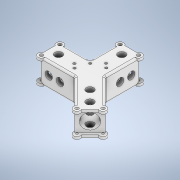
# Autodesk Inventor part: BracketV3
Saved by Autodesk Inventor 2022 (Build 260153000, 153)
## iProperties
Created: 2022-02-09
Part Number: BracketV3
Material: Generic
Document SubType Name: Modeling
Designer: ultra
Density: 1 g/cm^3
Appearance: Smooth - White
Author: ultra
Autodesk Inventor part; units mm, degrees
ref_plane "YZ Plane" through (0, 0, 0) normal (1, 0, 0) x (0, 1, 0)
ref_plane "XZ Plane" through (0, 0, 0) normal (0, 1, 0) x (-1, 0, 0)
ref_plane "XY Plane" through (0, 0, 0) normal (0, 0, 1) x (1, 0, 0)
sketch "Sketch1" plane through (0, 0, 0) normal (1, 0, 0) x (0, 1, 0)
  line L0 (0, 0) -> (41.5544, 0)
  line L1 (41.5544, 0) -> (41.5544, 37.0078)
  line L2 (41.5544, 37.0078) -> (0, 37.0078)
  line L3 (0, 37.0078) -> (0, 0)
  circle A0 centre (20.7772, 18.5039) radius 12.8778
  dimension "d0" = 41.5544
  dimension "d1" = 37.0078
  dimension "d2" = 25.7556
  constraints: 8 end point, 2 parallel, 1 centre point, 1 horizontal, 1 perpendicular
  measures "d0" distance of L2.end L1.end
  measures "d1" distance of L1.end L0.end
  measures "d2" diameter of A0
extrude "Extrusion1" add sketch "Sketch1" along normal blind 50.8
sketch "Sketch2" plane through (0, 0, 0) normal (0, 0, -1) x (-1, 0, 0)
  line L0 (-50.8, 0) -> (-50.8, 41.5544) projected
  line L1 (-50.8, 41.5544) -> (-87.8078, 41.5544)
  line L2 (-87.8078, 41.5544) -> (-87.8078, 0)
  line L3 (-87.8078, 0) -> (-50.8, 0)
  line L4 (-50.8, 0) -> (-50.8, 41.5544)
  circle A0 centre (-69.3039, 20.7772) radius 12.8778
  dimension "d5" = 37.0078
  dimension "d6" = 25.7556
  constraints: 8 end point, 2 parallel, 1 centre point, 1 horizontal, 1 perpendicular
  measures "d5" distance of L3.end L2.end
  measures "d6" diameter of A0
extrude "Extrusion2" add sketch "Sketch2" against normal up to surface (37.0078 mm away) contours L3 L2 L1 L0 | A0
sketch "Sketch3" plane through (0, 0, 0) normal (0, 0, -1) x (-1, 0, 0)
  line L0 (0, 41.5544) -> (-87.8078, 41.5544) projected
  line L1 (-87.8078, 41.5544) -> (-87.8078, 0) projected
  line L2 (0, 0) -> (-87.8078, 0) projected
  line L3 (0, 0) -> (-87.8078, 0) projected
  line L4 (-87.8078, 41.5544) -> (-50.8, 41.5544)
  line L5 (-50.8, 41.5544) -> (-50.8, 0)
  line L6 (-50.8, 0) -> (-87.8078, 0)
  line L7 (-87.8078, 0) -> (-87.8078, 41.5544)
  circle A0 centre (-69.3039, 20.7772) radius 12.8778
  point P0 (-50.8, 0)
  dimension "d9" = 37.0078
  dimension "d10" = 25.7556
  constraints: 8 end point, 2 parallel, 1 centre point, 1 horizontal, 1 perpendicular, 1 point on line
  measures "d9" distance of L5.end L6.end
  measures "d10" diameter of A0
extrude "Extrusion3" add sketch "Sketch3" along normal blind 50.8
sketch "Sketch4" plane through (0, 41.5544, 37.0078) normal (0, 1, 0) x (1, 0, 0)
  line L0 (0, 0) -> (87.8078, 0) projected
  line L1 (87.8078, 87.8078) -> (87.8078, 0) projected
  line L2 (50.8, 37.0078) -> (50.8, 87.8078) projected
  line L3 (87.8078, 0) -> (87.8078, 87.8078) projected
  line L4 (50.8, 37.0078) -> (87.8078, 0)
  line L5 (87.8078, 0) -> (123.1594, -36.4815)
  line L6 (87.8078, 0) -> (100.892, 13.0842)
  line L7 (0, 0) -> (87.8078, 0) projected
  line L8 (87.8078, 0) -> (74.7236, -13.0842)
  line L9 (100.892, 13.0842) -> (87.8078, 26.1685)
  line L10 (74.7236, -13.0842) -> (61.6393, 0)
  line L11 (100.892, 13.0842) -> (136.8086, -22.8323)
  line L12 (136.8086, -22.8323) -> (123.1594, -36.4815)
  line L13 (123.1594, -36.4815) -> (110.6401, -49.0008)
  line L14 (123.1594, -36.4815) -> (140.8643, -36.4815) construction
  line L15 (110.6401, -49.0008) -> (74.7236, -13.0842)
  dimension "d13" = 50.8
  dimension "d14" = 18.5039
  dimension "d15" = 18.5039
  dimension "d16" = 135
  constraints: 22 end point, 4 point on line, 3 perpendicular, 1 equal length, 1 horizontal
  measures "d13" distance of L0.end L5.end
  measures "d14" distance of L0.end L6.end
  measures "d15" distance of L0.end L8.end
  measures "d16" angle of L13 L14
extrude "Extrusion4" add sketch "Sketch4" against normal up to surface (41.5544 mm away)
sketch "Sketch5" plane through (136.8086, 0, 59.8401) normal (0.7071068, 0, 0.7071068) x (0.7071068, 0, -0.7071068)
  line L0 (-18.5039, 41.5544) -> (-18.5039, 0) projected
  circle A0 centre (-18.5039, 20.7772) radius 12.8778
  point P0 (-54.4249, 0)
  dimension "d19" = 25.7556
  constraints: 1 centre point, 1 midpoint
  measures "d19" diameter of A0
extrude "Extrusion5" cut sketch "Sketch5" against normal blind 76.2
sketch "Sketch6" plane through (0, 41.5544, 37.0078) normal (0, 1, 0) x (1, 0, 0)
  line L0 (0, 37.0078) -> (0, 0) projected
  line L1 (0, 0) -> (61.6393, 0) projected
  line L2 (61.6393, 0) -> (110.6401, -49.0008) projected
  line L3 (110.6401, -49.0008) -> (136.8086, -22.8323) projected
  line L4 (136.8086, -22.8323) -> (87.8078, 26.1685) projected
  line L5 (87.8078, 87.8078) -> (87.8078, 26.1685) projected
  line L6 (50.8, 87.8078) -> (87.8078, 87.8078) projected
  line L7 (50.8, 37.0078) -> (50.8, 87.8078) projected
  line L8 (0, 37.0078) -> (50.8, 37.0078) projected
  line L9 (0, 18.5039) -> (69.3039, 18.5039)
  line L10 (69.3039, 18.5039) -> (69.3039, 87.8078)
  line L11 (56.4261, 87.8078) -> (82.1817, 87.8078) projected
  line L12 (69.3039, 18.5039) -> (123.7244, -35.9166)
  circle A0 centre (2.4892, 2.879) radius 1.778
  circle A1 centre (2.4892, 34.1288) radius 1.778
  circle A2 centre (84.9288, 85.3186) radius 1.778
  circle A3 centre (53.679, 85.3186) radius 1.778
  circle A4 centre (110.9158, -45.2049) radius 1.778
  circle A5 centre (133.0127, -23.108) radius 1.778
  dimension "d22" = 3.556
  dimension "d23" = 3.556
  dimension "d24" = 2.4892
  dimension "d25" = 2.4892
  dimension "d26" = 2.879
  dimension "d27" = 2.879
  dimension "d28" = 3.556
  dimension "d29" = 3.556
  dimension "d30" = 2.4892
  dimension "d31" = 2.4892
  dimension "d32" = 2.879
  dimension "d33" = 2.879
  dimension "d34" = 3.556
  dimension "d35" = 3.556
  dimension "d36" = 2.4892
  dimension "d37" = 2.4892
  dimension "d38" = 2.879
  dimension "d39" = 2.879
  constraints: 6 centre point, 6 end point, 3 midpoint, 1 perpendicular
  measures "d22" diameter of A0
  measures "d23" diameter of A1
  measures "d24" distance from line of L0 A0.centre
  measures "d25" distance from line of L0 A1.centre
  measures "d26" distance from line of L1 A0.centre
  measures "d27" distance from line of L8 A1.centre
  measures "d28" diameter of A2
  measures "d29" diameter of A3
  measures "d30" vertical distance of L11.start A3.centre
  measures "d31" distance from line of L6 A2.centre
  measures "d32" distance from line of L5 A2.centre
  measures "d33" distance from line of L7 A3.centre
  measures "d34" diameter of A4
  measures "d35" diameter of A5
  measures "d36" distance from line of L3 A4.centre
  measures "d37" distance from line of L3 A5.centre
  measures "d38" distance from line of L4 A5.centre
  measures "d39" distance from line of L2 A4.centre
extrude "Extrusion6" cut sketch "Sketch6" against normal blind 50.8 contours A0 | A1 | A2 | A3 | A4 | A5
sketch "Sketch7" plane through (0, 41.5544, 37.0078) normal (0, 1, 0) x (1, 0, 0)
  circle A0 centre (2.4892, 2.879) radius 1.778 projected
  circle A1 centre (110.9158, -45.2049) radius 1.778 projected
  circle A2 centre (53.679, 85.3186) radius 1.778 projected
  circle A3 centre (2.4892, 34.1288) radius 1.778 projected
  circle A4 centre (84.9288, 85.3186) radius 1.778 projected
  line L0 (0, 37.0078) -> (0, 0) projected
  line L1 (0, 0) -> (61.6393, 0) projected
  line L2 (61.6393, 0) -> (110.6401, -49.0008) projected
  line L3 (110.6401, -49.0008) -> (136.8086, -22.8323) projected
  line L4 (136.8086, -22.8323) -> (87.8078, 26.1685) projected
  line L5 (87.8078, 87.8078) -> (87.8078, 26.1685) projected
  line L6 (50.8, 87.8078) -> (87.8078, 87.8078) projected
  line L7 (50.8, 37.0078) -> (50.8, 87.8078) projected
  line L8 (0, 37.0078) -> (50.8, 37.0078) projected
  circle A5 centre (133.0127, -23.108) radius 1.778 projected
  circle A6 centre (133.0127, -23.108) radius 6
  circle A7 centre (110.9158, -45.2049) radius 6
  circle A8 centre (2.4892, 2.879) radius 6
  circle A9 centre (2.4892, 34.1288) radius 6
  circle A10 centre (53.679, 85.3186) radius 6
  circle A11 centre (84.9288, 85.3186) radius 6
  point P0 (0, 8.3383)
  point P1 (7.7534, 0)
  point P2 (7.7534, 37.0078)
  point P3 (0, 28.6695)
  point P4 (59.1383, 87.8078)
  point P5 (50.8, 80.0544)
  point P6 (79.4695, 87.8078)
  point P7 (87.8078, 80.0544)
  point P8 (130.9126, -28.7284)
  point P9 (131.3262, -17.3499)
  point P10 (105.1577, -43.5184)
  point P11 (116.5362, -43.1048)
  dimension "d42" = 12
  dimension "d43" = 12
  dimension "d44" = 12
  dimension "d45" = 12
  dimension "d46" = 12
  dimension "d47" = 12
  constraints: 6 centre point, 6 coincident
  measures "d42" diameter of A6
  measures "d43" diameter of A7
  measures "d44" diameter of A8
  measures "d45" diameter of A9
  measures "d46" diameter of A10
  measures "d47" diameter of A11
extrude "Extrusion7" add sketch "Sketch7" against normal blind 4.7752 contours L0 A9 L8 | L0 L1 A8 | A10 L6 L7 | L2 L3 A7 | A11 L5 L6 | L3 L4 A6 picked at (-0.4033, 31.694) picked at (-0.4033, 5.3138) picked at (56.1138, 88.2111) picked at (106.9061, -45.8277) picked at (82.5067, 88.2271) picked at (133.3453, -26.876)
sketch "Sketch8" plane through (0, 0, 0) normal (0, -1, 0) x (1, 0, 0)
  circle A0 centre (2.4892, 34.1288) radius 1.778 projected
  circle A1 centre (53.679, -48.3108) radius 1.778 projected
  circle A2 centre (2.4892, 2.879) radius 1.778 projected
  circle A3 centre (84.9288, -48.3108) radius 1.778 projected
  line L0 (0, 37.0078) -> (0, 0) projected
  line L1 (0, 0) -> (50.8, 0) projected
  line L2 (50.8, 0) -> (50.8, -50.8) projected
  line L3 (87.8078, -50.8) -> (50.8, -50.8) projected
  line L4 (87.8078, 10.8393) -> (87.8078, -50.8) projected
  line L5 (136.8086, 59.8401) -> (87.8078, 10.8393) projected
  line L6 (110.6401, 86.0086) -> (136.8086, 59.8401) projected
  line L7 (61.6393, 37.0078) -> (110.6401, 86.0086) projected
  line L8 (0, 37.0078) -> (61.6393, 37.0078) projected
  circle A4 centre (110.9158, 82.2127) radius 1.778 projected
  circle A5 centre (110.9158, 82.2127) radius 6
  circle A6 centre (133.0127, 60.1158) radius 1.778 projected
  circle A7 centre (133.0127, 60.1158) radius 6
  circle A8 centre (84.9288, -48.3108) radius 6
  circle A9 centre (53.679, -48.3108) radius 6
  circle A10 centre (2.4892, 2.879) radius 6
  circle A11 centre (2.4892, 34.1288) radius 6
  point P0 (0, 8.3383)
  point P1 (7.7534, 0)
  point P2 (7.7534, 37.0078)
  point P3 (0, 28.6695)
  point P4 (116.5362, 80.1126)
  point P5 (105.1577, 80.5262)
  point P6 (131.3262, 54.3577)
  point P7 (130.9126, 65.7362)
  point P8 (87.8078, -43.0466)
  point P9 (79.4695, -50.8)
  point P10 (50.8, -43.0466)
  point P11 (59.1383, -50.8)
  dimension "d50" = 12
  constraints: 6 centre point, 6 coincident
  measures "d50" diameter of A5
extrude "Extrusion8" add sketch "Sketch8" against normal blind 4.7752 contours L0 A11 L8 | L0 L1 A10 | A5 L6 L7 | L2 L3 A9 | A7 L5 L6 | L3 L4 A8 picked at (-0.4033, 31.694) picked at (-0.4033, 5.3138) picked at (106.9061, 82.8355) picked at (56.1138, -51.2033) picked at (133.3453, 63.8838) picked at (82.5067, -51.2193)
sketch "Sketch9" plane through (0, 41.5544, 28.6695) normal (0, 1, 0) x (1, 0, 0)
  circle A0 centre (2.4892, -5.4593) radius 1.778 projected
  circle A1 centre (110.9158, -53.5432) radius 1.778 projected
  circle A2 centre (53.679, 76.9803) radius 1.778 projected
  circle A3 centre (2.4892, 25.7905) radius 1.778 projected
  circle A4 centre (133.0127, -31.4463) radius 1.778 projected
  circle A5 centre (84.9288, 76.9803) radius 1.778 projected
  arc A6 (0, 0) -> (7.7534, -8.3383) centre (2.4892, -5.4593) ccw projected
  arc A7 (105.1577, -51.8567) -> (116.5362, -51.443) centre (110.9158, -53.5432) ccw projected
  arc A8 (87.8078, 71.7161) -> (79.4695, 79.4695) centre (84.9288, 76.9803) ccw projected
  arc A9 (7.7534, 28.6695) -> (0, 20.3312) centre (2.4892, 25.7905) ccw projected
  circle A10 centre (110.9158, -53.5432) radius 2.95
  circle A11 centre (133.0127, -31.4463) radius 1.778 projected
  circle A12 centre (133.0127, -31.4463) radius 2.95
  circle A13 centre (84.9288, 76.9803) radius 2.95
  circle A14 centre (53.679, 76.9803) radius 1.778 projected
  circle A15 centre (53.679, 76.9803) radius 2.95
  circle A16 centre (2.4892, 25.7905) radius 2.95
  circle A17 centre (2.4892, -5.4593) radius 2.95
  point P0 (0, 28.6695)
  dimension "d53" = 5.9
  dimension "d54" = 5.9
  dimension "d55" = 5.9
  dimension "d56" = 5.9
  dimension "d57" = 5.9
  dimension "d58" = 5.9
  constraints: 6 centre point, 6 coincident
  measures "d53" diameter of A10
  measures "d54" diameter of A12
  measures "d55" diameter of A13
  measures "d56" diameter of A15
  measures "d57" diameter of A16
  measures "d58" diameter of A17
sketch "Sketch10" plane through (0, 0, -50.8) normal (0, 0, -1) x (-1, 0, 0)
  line L0 (-59.1383, 4.7752) -> (-50.8, 4.7752) projected
  line L1 (-50.8, 4.7752) -> (-50.8, 36.7792) projected
  line L2 (-50.8, 36.7792) -> (-59.1383, 36.7792) projected
  line L3 (-79.4695, 36.7792) -> (-87.8078, 36.7792) projected
  line L4 (-87.8078, 36.7792) -> (-87.8078, 4.7752) projected
  line L5 (-87.8078, 4.7752) -> (-79.4695, 4.7752) projected
  circle A0 centre (-69.3039, 20.7772) radius 12.8778 projected
  line L6 (-87.8078, 4.7752) -> (-50.8, 4.7752)
  line L7 (-50.8, 4.7752) -> (-50.8, 36.7792)
  line L8 (-50.8, 36.7792) -> (-87.8078, 36.7792)
  line L9 (-87.8078, 36.7792) -> (-87.8078, 4.7752)
  line L10 (-87.8078, 4.7752) -> (-50.8, 36.7792) construction
  line L11 (-50.8, 4.7752) -> (-87.8078, 36.7792) construction
  point P0 (0, 0)
  constraints: 12 end point, 2 midpoint, 2 parallel, 1 horizontal, 1 perpendicular
extrude "Extrusion9" cut sketch "Sketch10" against normal blind 5.0038
sketch "Sketch11" plane through (0, 0, 0) normal (-1, 0, 0) x (0, 0, 1)
  line L0 (28.6695, 4.7752) -> (37.0078, 4.7752) projected
  line L1 (37.0078, 36.7792) -> (37.0078, 4.7752) projected
  line L2 (37.0078, 36.7792) -> (28.6695, 36.7792) projected
  line L3 (8.3383, 36.7792) -> (0, 36.7792) projected
  line L4 (0, 4.7752) -> (0, 36.7792) projected
  line L5 (0, 4.7752) -> (8.3383, 4.7752) projected
  circle A0 centre (18.5039, 20.7772) radius 12.8778 projected
  line L6 (0, 4.7752) -> (37.0078, 4.7752)
  line L7 (37.0078, 4.7752) -> (37.0078, 36.7792)
  line L8 (37.0078, 36.7792) -> (0, 36.7792)
  line L9 (0, 36.7792) -> (0, 4.7752)
  line L10 (0, 4.7752) -> (37.0078, 36.7792) construction
  line L11 (37.0078, 4.7752) -> (0, 36.7792) construction
  point P0 (0, 0)
  constraints: 12 end point, 2 midpoint, 2 parallel, 1 horizontal, 1 perpendicular
extrude "Extrusion10" cut sketch "Sketch11" against normal blind 5.0038
sketch "Sketch12" plane through (130.9126, 36.7792, 65.7362) normal (0.7071068, 0, 0.7071068) x (0.7071068, 0, -0.7071068)
  line L0 (0, -32.004) -> (8.3383, -32.004) projected
  line L1 (8.3383, 0) -> (8.3383, -32.004) projected
  line L2 (8.3383, 0) -> (0, 0) projected
  line L3 (-20.3312, 0) -> (-28.6695, 0) projected
  line L4 (-28.6695, 0) -> (-28.6695, -32.004) projected
  line L5 (-28.6695, -32.004) -> (-20.3312, -32.004) projected
  circle A0 centre (-10.1656, -16.002) radius 12.8778 projected
  line L6 (-28.6695, -32.004) -> (8.3383, -32.004)
  line L7 (8.3383, -32.004) -> (8.3383, 0)
  line L8 (8.3383, 0) -> (-28.6695, 0)
  line L9 (-28.6695, 0) -> (-28.6695, -32.004)
  line L10 (-28.6695, -32.004) -> (8.3383, 0) construction
  line L11 (8.3383, -32.004) -> (-28.6695, 0) construction
  point P0 (-46.0866, -36.7792)
  point P1 (-20.3312, 0)
  point P2 (-20.3312, -32.004)
  constraints: 12 end point, 2 midpoint, 2 parallel, 1 horizontal, 1 perpendicular
extrude "Extrusion11" cut sketch "Sketch12" against normal blind 5.0038
extrude "Extrusion12" cut sketch "Sketch9" against normal blind 5.08
fillet "Fillet1" radius 3.175 15 edges at (50.8, 20.7772, 0) (29.2767, 41.5544, 0) (50.8, 41.5544, -21.5233) (50.8, 0, -21.5233) (29.2767, 0, 0) (34.6963, 41.5544, 37.0078) (83.3985, 41.5544, 58.767) (83.3985, 0, 58.767) (109.567, 41.5544, 32.5985) (109.567, 0, 32.5985) (87.8078, 41.5544, -16.1037) (87.8078, 0, -16.1037) (34.6963, 0, 37.0078) (61.6393, 20.7772, 37.0078) (87.8078, 20.7772, 10.8393)
sketch "Sketch15" plane through (0, 0, 8.3383) normal (0, -1, 0) x (1, 0, 0)
  line L0 (0, 0) -> (0, 20.3312) projected
  line L1 (116.755, -37.314) -> (68.3935, 11.0475)
  line L2 (68.3935, 11.0475) -> (118.0223, 60.6763)
  line L3 (68.3935, 11.0475) -> (18.7646, 60.6763) construction
  line L4 (73.5122, 12.7537) -> (70.0997, 16.1662)
  line L5 (70.0997, 16.1662) -> (63.2747, 9.3412)
  line L6 (63.2747, 9.3412) -> (66.6872, 5.9287)
  line L7 (66.6872, 5.9287) -> (73.5122, 12.7537)
  line L8 (73.5122, 12.7537) -> (63.2747, 9.3412) construction
  line L9 (70.0997, 16.1662) -> (66.6872, 5.9287) construction
  line L10 (78.0024, 12.7537) -> (70.0997, 20.6564)
  line L11 (70.0997, 20.6564) -> (58.7846, 9.3412)
  line L12 (58.7846, 9.3412) -> (66.6872, 1.4386)
  line L13 (66.6872, 1.4386) -> (78.0024, 12.7537)
  line L14 (78.0024, 12.7537) -> (58.7846, 9.3412) construction
  line L15 (70.0997, 20.6564) -> (66.6872, 1.4386) construction
  point P0 (0, -8.3383)
  dimension "d104" = 90
  dimension "d105" = 4.826
  dimension "d106" = 9.652
  dimension "d107" = 11.176
  dimension "d108" = 16.002
  constraints: 30 end point, 4 midpoint, 4 parallel, 3 perpendicular
  measures "d104" angle of L2 L3
  measures "d105" distance of L6.end L5.end
  measures "d106" distance of L5.end L4.end
  measures "d107" distance of L12.end L11.end
  measures "d108" distance of L11.end L10.end
extrude "Extrusion14" add sketch "Sketch15" along normal blind 12.7 contours L13 L12 L11 L10 L2 L4 L5 L6 L7 L1 | L1 L7 L4 L2 L10 L13
sketch "Sketch16" plane through (58.7846, 0, 17.6795) normal (-0.7071068, 0, 0.7071068) x (0.7071068, 0, 0.7071068)
  line L0 (0, 0) -> (0, -12.7) projected
  line L1 (16.002, -12.7) -> (0, -12.7) projected
  circle A0 centre (8.001, -7.112) radius 3.175
  point P0 (-54.0683, 0)
  dimension "d111" = 6.35
  dimension "d112" = 8.001
  dimension "d113" = 5.588
  constraints: 1 centre point
  measures "d111" diameter of A0
  measures "d112" distance from line of L0 A0.centre
  measures "d113" distance from line of A0.centre L1
extrude "Extrusion15" cut sketch "Sketch16" against normal blind 279.4
sketch "Sketch18" plane through (0, 41.5544, 28.6695) normal (0, 1, 0) x (1, 0, 0)
  circle A0 centre (76.2759, 30.7551) radius 2.159
  circle A1 centre (69.4016, 37.3483) radius 2.159
  circle A2 centre (55.9312, 23.8779) radius 2.159
  circle A3 centre (42.7448, 10.1294) radius 2.159
  circle A4 centre (49.6191, 3.5362) radius 2.159
  point P0 (0, 28.6695)
  dimension "d149" = 4.318
  dimension "d150" = 4.318
  dimension "d151" = 4.318
  dimension "d152" = 4.318
  dimension "d153" = 4.318
  constraints: 5 centre point
  measures "d149" diameter of A0
  measures "d150" diameter of A1
  measures "d151" diameter of A2
  measures "d152" diameter of A3
  measures "d153" diameter of A4
fillet "Fillet2" radius 6.35 4 edges at (62.7359, 0, 13.7282) (72.3448, 0, 15.4345) (74.051, 0, 25.0433) (64.4422, 0, 23.3371)
fillet "Fillet3" radius 3.175 8 edges at (66.6872, -1.8599, 7.1467) (66.6872, -9.525, 9.7769) (80.6326, -1.8599, 21.092) (78.0024, -9.525, 21.092) (70.0997, -1.8599, 31.6249) (70.0997, -9.525, 28.9947) (56.1544, -1.8599, 17.6795) (58.7846, -9.525, 17.6795)
sketch "Sketch20" plane through (0, 36.7792, 37.0078) normal (0, -1, 0) x (1, 0, 0)
  arc A0 (5.0038, -1.3365) -> (5.0038, -4.4215) centre (2.4892, -2.879) ccw projected
  line L0 (5.0038, -1.3365) -> (5.0038, 0) projected
  line L1 (7.7534, 0) -> (5.0038, 0) projected
  arc A1 (7.7534, 0) -> (0, -8.3383) centre (2.4892, -2.879) ccw projected
  line L2 (0, -28.6695) -> (0, -8.3383) projected
  arc A2 (0, -28.6695) -> (7.7534, -37.0078) centre (2.4892, -34.1288) ccw projected
  line L3 (5.0038, -37.0078) -> (7.7534, -37.0078) projected
  line L4 (5.0038, -37.0078) -> (5.0038, -35.6713) projected
  arc A3 (5.0038, -32.5863) -> (5.0038, -35.6713) centre (2.4892, -34.1288) ccw projected
  line L5 (5.0038, -32.5863) -> (5.0038, -4.4215) projected
  point P0 (0, -37.0078)
extrude "Extrusion19" cut sketch "Sketch20" against normal blind 0.381
sketch "Sketch21" plane through (0, 4.7752, 0) normal (0, 1, 0) x (1, 0, 0)
  circle A0 centre (2.4892, -34.1288) radius 1.5875 projected
  circle A1 centre (2.4892, -2.879) radius 1.5875 projected
  line L0 (7.7534, 0) -> (5.0038, 0) projected
  arc A2 (7.7534, 0) -> (0, -8.3383) centre (2.4892, -2.879) ccw projected
  line L1 (0, -28.6695) -> (0, -8.3383) projected
  arc A3 (0, -28.6695) -> (7.7534, -37.0078) centre (2.4892, -34.1288) ccw projected
  line L2 (5.0038, -37.0078) -> (7.7534, -37.0078) projected
  line L3 (5.0038, -37.0078) -> (5.0038, 0) projected
  point P0 (0, 0)
extrude "Extrusion20" cut sketch "Sketch21" against normal blind 0.381
sketch "Sketch22" plane through (0, 4.7752, 0) normal (0, 1, 0) x (1, 0, 0)
  circle A0 centre (53.679, 48.3108) radius 1.5875 projected
  circle A1 centre (84.9288, 48.3108) radius 1.5875 projected
  line L0 (87.8078, 43.0466) -> (87.8078, 45.7962) projected
  arc A2 (87.8078, 43.0466) -> (79.4695, 50.8) centre (84.9288, 48.3108) ccw projected
  line L1 (59.1383, 50.8) -> (79.4695, 50.8) projected
  arc A3 (59.1383, 50.8) -> (50.8, 43.0466) centre (53.679, 48.3108) ccw projected
  line L2 (50.8, 45.7962) -> (50.8, 43.0466) projected
  line L3 (50.8, 45.7962) -> (87.8078, 45.7962) projected
  point P0 (0, 0)
extrude "Extrusion21" cut sketch "Sketch22" against normal blind 0.381
sketch "Sketch23" plane through (0, 4.7752, 0) normal (0, 1, 0) x (1, 0, 0)
  circle A0 centre (110.9158, -82.2127) radius 1.5875 projected
  circle A1 centre (133.0127, -60.1158) radius 1.5875 projected
  line L0 (105.1577, -80.5262) -> (107.1019, -82.4704) projected
  arc A2 (105.1577, -80.5262) -> (116.5362, -80.1126) centre (110.9158, -82.2127) ccw projected
  line L1 (130.9126, -65.7362) -> (116.5362, -80.1126) projected
  arc A3 (130.9126, -65.7362) -> (131.3262, -54.3577) centre (133.0127, -60.1158) ccw projected
  line L2 (133.2704, -56.3019) -> (131.3262, -54.3577) projected
  line L3 (133.2704, -56.3019) -> (107.1019, -82.4704) projected
  point P0 (0, 0)
extrude "Extrusion22" cut sketch "Sketch23" against normal blind 0.381
sketch "Sketch24" plane through (0, 36.7792, 37.0078) normal (0, -1, 0) x (1, 0, 0)
  arc A0 (52.1365, -82.804) -> (55.2215, -82.804) centre (53.679, -85.3186) ccw projected
  line L0 (52.1365, -82.804) -> (50.8, -82.804) projected
  line L1 (50.8, -80.0544) -> (50.8, -82.804) projected
  arc A1 (50.8, -80.0544) -> (59.1383, -87.8078) centre (53.679, -85.3186) ccw projected
  line L2 (79.4695, -87.8078) -> (59.1383, -87.8078) projected
  arc A2 (79.4695, -87.8078) -> (87.8078, -80.0544) centre (84.9288, -85.3186) ccw projected
  line L3 (87.8078, -82.804) -> (87.8078, -80.0544) projected
  line L4 (87.8078, -82.804) -> (86.4713, -82.804) projected
  arc A3 (83.3863, -82.804) -> (86.4713, -82.804) centre (84.9288, -85.3186) ccw projected
  line L5 (83.3863, -82.804) -> (55.2215, -82.804) projected
  point P0 (0, -37.0078)
extrude "Extrusion23" cut sketch "Sketch24" against normal blind 0.381
sketch "Sketch25" plane through (0, 36.7792, 37.0078) normal (0, -1, 0) x (1, 0, 0)
  arc A0 (110.2284, 42.3361) -> (108.047, 44.5175) centre (110.9158, 45.2049) ccw projected
  line L0 (110.2284, 42.3361) -> (130.1439, 22.4206) projected
  arc A1 (132.3253, 20.2392) -> (130.1439, 22.4206) centre (133.0127, 23.108) ccw projected
  line L1 (132.3253, 20.2392) -> (133.2704, 19.2941) projected
  line L2 (131.3262, 17.3499) -> (133.2704, 19.2941) projected
  arc A2 (131.3262, 17.3499) -> (130.9126, 28.7284) centre (133.0127, 23.108) ccw projected
  line L3 (116.5362, 43.1048) -> (130.9126, 28.7284) projected
  arc A3 (116.5362, 43.1048) -> (105.1577, 43.5184) centre (110.9158, 45.2049) ccw projected
  line L4 (107.1019, 45.4626) -> (105.1577, 43.5184) projected
  line L5 (107.1019, 45.4626) -> (108.047, 44.5175) projected
  point P0 (0, -37.0078)
extrude "Extrusion24" cut sketch "Sketch25" against normal blind 0.381
extrude "Extrusion25" cut sketch "Sketch18" against normal blind 9.525
sketch "Sketch27" plane through (62.5693, 3.175, 37.9377) normal (-0.7071068, 0, 0.7071068) x (0.7071068, 0, 0.7071068)
  line L0 (62.9787, 1.2192) -> (62.9787, 33.9852) projected
  line L1 (0, 0) -> (0, 35.2044) projected
  line L2 (62.9787, 33.9852) -> (62.9787, 1.2192) projected
  line L3 (62.9787, 17.6022) -> (0, 17.6022)
  circle A0 centre (50.2787, 17.6022) radius 6.35
  circle A1 centre (24.8787, 17.6022) radius 6.35
  point P0 (-71.0692, -3.175)
  dimension "d162" = 12.7
  dimension "d163" = 12.7
  dimension "d166" = 25.4
  constraints: 2 centre point, 2 end point, 2 midpoint, 1 horizontal, 1 point on line, 2 other
  measures "d162" diameter of A0
  measures "d163" distance from line of L0 A0.centre
  measures "d166" distance of A0.centre A1.centre
extrude "Extrusion27" cut sketch "Sketch27" against normal blind 76.2
sketch "Sketch28" plane through (7.7534, 3.175, 37.0078) normal (0, 0, 1) x (1, 0, 0)
  line L0 (52.5708, 35.2044) -> (52.5708, 0) projected
  line L1 (-2.7496, 33.9852) -> (-2.7496, 1.2192) projected
  line L2 (-2.7496, 30.48) -> (-2.7496, 4.7244) projected
  line L3 (-2.7496, 17.6022) -> (52.9835, 17.6022)
  ellipse E0 centre (62.0895, 17.6022) end of major axis (62.0895, 4.7244) minor radius 9.106 projected
  circle A0 centre (9.9504, 17.6022) radius 6.35
  circle A1 centre (29.0004, 17.6022) radius 6.35
  point P0 (-7.7534, -3.175)
  dimension "d173" = 12.7
  dimension "d174" = 12.7
  dimension "d177" = 19.05
  constraints: 2 centre point, 2 end point, 1 horizontal, 1 horizontal alignment, 1 midpoint, 1 perpendicular, 1 point on line, 3 other
  measures "d173" diameter of A0
  measures "d174" distance from line of L1 A0.centre
  measures "d177" distance of A0.centre A1.centre
extrude "Extrusion28" cut sketch "Sketch28" against normal blind 76.2 contours A0 L3 | L3 A0 | A1 L3 | L3 A1
sketch "Sketch29" plane through (50.8, 3.175, -3.175) normal (-1, 0, 0) x (0, 0, 1)
  line L0 (0, 0) -> (-39.8716, 0) projected
  line L1 (-42.6212, 33.9852) -> (-42.6212, 1.2192) projected
  circle A0 centre (-29.9212, 17.6022) radius 6.35
  circle A1 centre (-10.8712, 17.6022) radius 6.35
  point P0 (3.175, -3.175)
  dimension "d184" = 12.7
  dimension "d185" = 12.7
  dimension "d188" = 19.05
  constraints: 2 centre point, 1 horizontal, 2 other
  measures "d184" diameter of A0
  measures "d185" distance from line of L1 A0.centre
  measures "d188" distance of A0.centre A1.centre
extrude "Extrusion29" cut sketch "Sketch29" against normal blind 76.2
sketch "Sketch31" plane through (0, 41.5544, 28.6695) normal (0, 1, 0) x (1, 0, 0)
  line L0 (53.975, 31.8445) -> (53.975, 70.9876) projected
  arc A0 (47.625, 25.4945) -> (53.975, 31.8445) centre (47.625, 31.8445) ccw projected
  line L1 (0, 20.3312) -> (0, 0) projected
  line L2 (116.5362, -51.443) -> (130.9126, -37.0667) projected
  line L3 (123.7244, -44.2549) -> (52.1151, 27.3544)
  line L4 (79.4695, 79.4695) -> (59.1383, 79.4695) projected
  line L5 (69.3039, 79.4695) -> (69.3039, 10.1656)
  line L6 (69.3039, 10.1656) -> (0, 10.1656)
  line L7 (69.3039, 79.4695) -> (69.3039, 66.7695)
  line L8 (69.3039, 66.7695) -> (76.9747, 66.7695)
  line L9 (69.3039, 66.7695) -> (61.6331, 66.7695)
  circle A1 centre (76.9747, 66.7695) radius 2.54
  circle A2 centre (61.6331, 66.7695) radius 2.54
  circle A3 centre (61.6331, 47.7195) radius 2.54
  circle A4 centre (76.9747, 47.7195) radius 2.54
  line L10 (123.7244, -44.2549) -> (114.7441, -35.2746)
  line L11 (114.7441, -35.2746) -> (120.1682, -29.8505)
  line L12 (120.1682, -29.8505) -> (114.7441, -35.2746)
  line L13 (114.7441, -35.2746) -> (109.3201, -40.6987)
  line L14 (0, 10.1656) -> (12.7, 10.1656)
  line L15 (12.7, 10.1656) -> (12.7, 2.4948)
  line L16 (12.7, 2.4948) -> (12.7, 10.1656)
  line L17 (12.7, 10.1656) -> (12.7, 17.8364)
  circle A5 centre (12.7, 2.4948) radius 2.54
  circle A6 centre (12.7, 17.8364) radius 2.54
  circle A7 centre (109.3201, -40.6987) radius 2.54
  circle A8 centre (120.1682, -29.8505) radius 2.54
  circle A9 centre (31.75, 17.8364) radius 2.54
  circle A10 centre (31.75, 2.4948) radius 2.54
  circle A11 centre (106.6978, -16.3802) radius 2.54
  circle A12 centre (95.8497, -27.2283) radius 2.54
  circle A13 centre (93.2274, -2.9098) radius 2.54
  circle A14 centre (82.3793, -13.7579) radius 2.54
  point P0 (0, 28.6695)
  dimension "d195" = 12.7
  dimension "d196" = 7.6708
  dimension "d197" = 7.6708
  dimension "d198" = 5.08
  dimension "d199" = 5.08
  dimension "d202" = 19.05
  dimension "d207" = 12.7
  dimension "d208" = 7.6708
  dimension "d209" = 7.6708
  dimension "d210" = 12.7
  dimension "d211" = 7.6708
  dimension "d212" = 7.6708
  dimension "d213" = 5.08
  dimension "d214" = 5.08
  dimension "d215" = 5.08
  dimension "d216" = 5.08
  dimension "d219" = 19.05
  dimension "d226" = 19.05
  constraints: 28 end point, 14 centre point, 6 coincident, 5 point on line, 3 horizontal, 3 midpoint, 2 collinear, 2 vertical, 1 perpendicular, 1 point on circle, 17 other
  measures "d195" distance of L5.start L7.end
  measures "d196" distance of L7.end L8.end
  measures "d197" distance of L7.end L9.end
  measures "d198" diameter of A1
  measures "d199" diameter of A2
  measures "d202" distance of A2.centre A3.centre
  measures "d207" distance of L3.start L10.end
  measures "d208" distance of L10.end L11.end
  measures "d209" distance of L10.end L13.end
  measures "d210" distance of L6.end L14.end
  measures "d211" distance of L14.end L15.end
  measures "d212" distance of L14.end L17.end
  measures "d213" diameter of A5
  measures "d214" diameter of A6
  measures "d215" diameter of A7
  measures "d216" diameter of A8
  measures "d219" distance of A6.centre A9.centre
  measures "d226" distance of A8.centre A11.centre
extrude "Extrusion30" [suppressed]
sketch "Sketch32" plane through (0, 0, 8.3383) normal (0, -1, 0) x (1, 0, 0)
  arc A0 (79.4695, -59.1383) -> (84.6328, -50.6564) centre (84.9288, -56.6491) ccw projected
  arc A1 (128.5659, 47.7493) -> (130.9126, 57.3979) centre (133.0127, 51.7775) ccw projected
  line L0 (116.5362, 71.7743) -> (130.9126, 57.3979) projected
  arc A2 (116.5362, 71.7743) -> (106.8876, 69.4277) centre (110.9158, 73.8744) ccw projected
  arc A3 (8.4819, 25.4945) -> (0, 20.3312) centre (2.4892, 25.7905) ccw projected
  line L1 (0, 20.3312) -> (0, 0) projected
  arc A4 (0, 0) -> (8.4819, -5.1633) centre (2.4892, -5.4593) ccw projected
  arc A5 (53.975, -50.6564) -> (59.1383, -59.1383) centre (53.679, -56.6491) ccw projected
  line L2 (79.4695, -59.1383) -> (59.1383, -59.1383) projected
  arc A6 (116.5362, 71.7743) -> (106.8876, 69.4277) centre (110.9158, 73.8744) ccw projected
  line L3 (115.3626, 77.9026) -> (137.2544, 56.0211)
  arc A7 (128.5659, 47.7493) -> (130.9126, 57.3979) centre (133.0127, 51.7775) ccw projected
  line L4 (84.9288, -62.6491) -> (53.679, -62.6491)
  line L5 (-3.297, 24.203) -> (-3.297, -3.8718)
  arc A8 (0, 0) -> (8.4819, -5.1633) centre (2.4892, -5.4593) ccw projected
  point P0 (0, -8.3383)
  point P1 (-3.297, -3.8718)
  point P2 (137.2544, 56.0211)
  constraints: 6 end point, 6 point on circle, 2 tangent, 1 perpendicular
extrude "Extrusion31" [suppressed]
fillet "Fillet4" [suppressed]
fillet "Fillet5" [suppressed]
sketch "Sketch33" plane through (0, 41.5544, 28.6695) normal (0, 1, 0) x (1, 0, 0)
  arc A0 (84.6328, 70.9876) -> (79.4695, 79.4695) centre (84.9288, 76.9803) ccw projected
  line L0 (59.1383, 79.4695) -> (79.4695, 79.4695) projected
  arc A1 (59.1383, 79.4695) -> (53.975, 70.9876) centre (53.679, 76.9803) ccw projected
  arc A2 (8.4819, 25.4945) -> (0, 20.3312) centre (2.4892, 25.7905) ccw projected
  line L1 (0, 20.3312) -> (0, 0) projected
  arc A3 (0, 0) -> (8.4819, -5.1633) centre (2.4892, -5.4593) ccw projected
  arc A4 (106.8876, -49.0964) -> (116.5362, -51.443) centre (110.9158, -53.5432) ccw projected
  line L2 (116.5362, -51.443) -> (130.9126, -37.0667) projected
  arc A5 (130.9126, -37.0667) -> (128.5659, -27.4181) centre (133.0127, -31.4463) ccw projected
  arc A6 (0, 0) -> (7.7534, -8.3383) centre (2.4892, -5.4593) ccw projected
  line L3 (-3.5108, -5.4593) -> (-3.5108, 27.3544)
  line L4 (84.9288, 82.9803) -> (53.679, 82.9803)
  arc A7 (105.1577, -51.8567) -> (116.5362, -51.443) centre (110.9158, -53.5432) ccw projected
  line L5 (114.5098, -58.3477) -> (137.2472, -35.697)
  point P0 (0, 28.6695)
  point P1 (-3.5108, 25.7905)
  point P2 (-3.5108, -5.4593)
  point P3 (115.7065, -57.1556)
  constraints: 6 end point, 5 point on circle, 2 tangent, 1 horizontal, 1 vertical
extrude "Extrusion32" [suppressed]
fillet "Fillet6" [suppressed]
sketch "Sketch34" plane through (0, 41.5544, 28.6695) normal (0, 1, 0) x (1, 0, 0)
  line L0 (59.1383, 79.4695) -> (79.4695, 79.4695) projected
  line L1 (0, 20.3312) -> (0, 0) projected
  line L2 (0, 10.1656) -> (69.8428, 9.6267)
  line L3 (78.9488, 18.7326) -> (60.7369, 0.5207) projected
  line L4 (69.8428, 9.6267) -> (123.7244, -44.2549)
  line L5 (116.5362, -51.443) -> (130.9126, -37.0667) projected
  line L6 (69.8428, 9.6267) -> (69.8428, 79.4695)
  line L7 (79.4695, 79.4695) -> (59.1383, 79.4695) projected
  circle A0 centre (15.875, 10.0431) radius 6.35
  circle A1 centre (69.8428, 63.5945) radius 6.35
  circle A2 centre (112.4991, -33.0296) radius 6.35
  circle A3 centre (94.5385, -15.069) radius 6.35
  point P0 (0, 28.6695)
  dimension "d240" = 12.7
  dimension "d241" = 12.7
  dimension "d242" = 12.7
  dimension "d243" = 15.875
  dimension "d244" = 15.875
  dimension "d247" = 25.4
  dimension "d254" = 15.875
  constraints: 6 end point, 4 centre point, 4 point on line, 3 midpoint, 1 perpendicular, 3 other
  measures "d240" diameter of A0
  measures "d241" diameter of A1
  measures "d242" diameter of A2
  measures "d243" distance from line of L1 A0.centre
  measures "d244" distance from line of L0 A1.centre
  measures "d247" distance of A2.centre A3.centre
  measures "d254" distance from line of L5 A2.centre
extrude "Extrusion33" cut sketch "Sketch34" against normal blind 50.8
equation "\"d7\" = d6"
body "Solid1"
